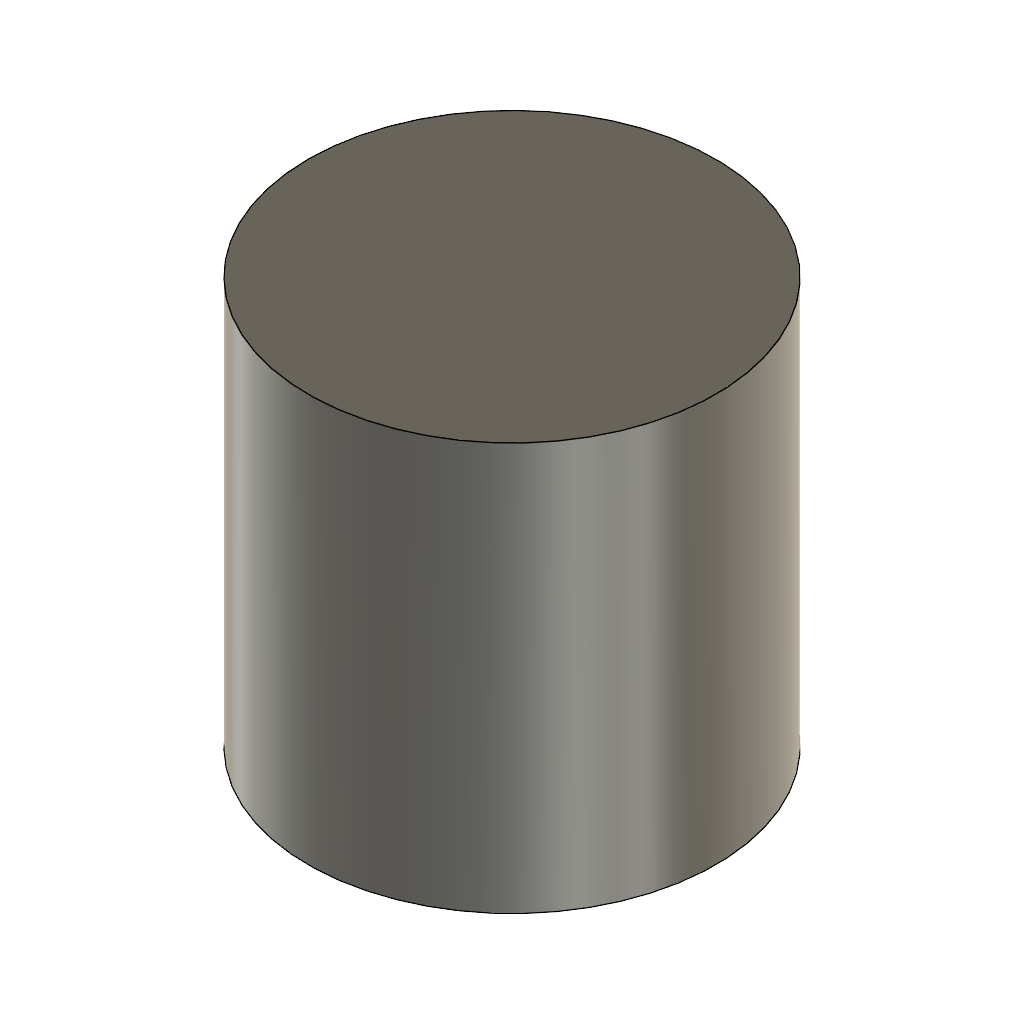
eleclinet-piezo-barrel (Autodesk Fusion 360 design; units mm, degrees)
Autodesk Fusion 360 part; units mm, degrees
sketch "Piezo-Shell-Circle" plane through (0, 0, 0) normal (0, 0, 1) x (1, 0, 0)
  circle A0 centre (0, 0) radius 7.5
  dimension "d1" = 15
  measures "d1" diameter of A0
extrude "Extrude1" add sketch "Piezo-Shell-Circle" along normal blind 15
shell "Shell1" thickness 1 removed faces 1 at (1.9158, 2.8099, 0)
ref_plane "WorkPlane1" through (0, 7.5, 5.2769) normal (0, 1, 0) x (1, 0, 0)
sketch "Sketch4" plane through (0, 7.5, 0) normal (0, 1, 0) x (1, 0, 0)
  line L0 (3, -13) -> (-3, -13)
  line L1 (-3, -13) -> (-3, -11)
  line L2 (-3, -11) -> (3, -11)
  line L3 (3, -11) -> (3, -13)
  dimension "d13" = 2
  dimension "d14" = 3
  dimension "d15" = 11
  dimension "d16" = 6
  constraint horizontal L0
  constraint vertical L1
  constraint horizontal L2
  constraint vertical L3
  measures "d13" distance of L0 L2
  measures "d14" distance of origin L1
  measures "d15" distance of origin L2
  measures "d16" distance of L1 L3
extrude "Extrude3" cut sketch "Sketch4" against normal blind 10
ref_plane "WorkPlane2" through (0, 0, 3.5) normal (0, 0, 1) x (1, 0, 0)
sketch "Sketch5" plane through (0, 0, 3.5) normal (0, 0, 1) x (1, 0, 0)
  circle A0 centre (0, 0) radius 7.5
  circle A1 centre (0, 0) radius 6
  dimension "d21" = 1.5
  dimension "d22" = 12
  constraint coincident A0.centre A1.centre
  constraint concentric A0 A1
  measures "d21" distance of A0 A1
  measures "d22" diameter of A1
extrude "Extrude4" add sketch "Sketch5" along normal blind 1
named bodies: "Piezo-Shell"
